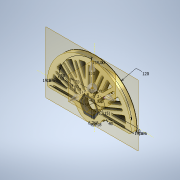
# Autodesk Inventor part: Capstonradialdisc_v2
Saved by Autodesk Inventor 2022 (Build 260153000, 153)
## iProperties
Created: 2022-03-11
Part Number: Capstonradialdisc_v2
Material: Generisch
Document SubType Name: Modeling
Designer: 123St
Density: 1 g/cm^3
Appearance: Gold - Metall
Mass: 270.626 g
Surface Area: 814.649 cm^2
Volume: 270.626 cm^3
CapstonDisc_Thickness: 16,000 mm
CapstonBig_Radius: 120,000 mm
Author: 123St
Autodesk Inventor part; units mm, degrees
ref_plane "YZ Plane" through (0, 0, 0) normal (1, 0, 0) x (0, 1, 0)
ref_plane "XZ Plane" through (0, 0, 0) normal (0, 1, 0) x (-1, 0, 0)
ref_plane "XY Plane" through (0, 0, 0) normal (0, 0, 1) x (1, 0, 0)
sketch "Skizze1" plane through (0, 0, 0) normal (0, 0, 1) x (1, 0, 0)
  line L0 (-4, 29) -> (4, 29)
  line L1 (4, 29) -> (4, 19.5959)
  line L2 (-4, 19.5959) -> (-4, 29)
  line L3 (-4, 29) -> (4, 19.5959) construction
  line L4 (4, 29) -> (-4, 19.5959) construction
  line L5 (0, 152) -> (0, -72) construction
  line L6 (-168, 0) -> (168, 0) construction
  line L7 (-40, 0) -> (-100, 0) construction
  line L8 (-40, -3) -> (-100, -3)
  line L9 (-100, 3) -> (-40, 3)
  arc A0 (-40, -3) -> (-40, 3) centre (-40, 0) ccw
  arc A1 (-100, 3) -> (-100, -3) centre (-100, 0) ccw
  arc A2 (-38.7298, -10) -> (38.7298, -10) centre (0, 0) ccw
  line L10 (-38.7298, -10) -> (-119.5826, -10)
  line L11 (38.7298, -10) -> (119.5826, -10)
  arc A3 (119.5826, -10) -> (-119.5826, -10) centre (0, 0) ccw
  arc A4 (-38.1032, 12.5357) -> (-35.8071, 18.079) centre (-36.9552, 15.3073) ccw
  line L12 (-91.2399, 41.04) -> (-35.8071, 18.079)
  line L13 (-36.9552, 15.3073) -> (-92.388, 38.2683) construction
  arc A5 (-91.2399, 41.04) -> (-93.536, 35.4967) centre (-92.388, 38.2683) ccw
  line L14 (-38.1032, 12.5357) -> (-93.536, 35.4967)
  arc A6 (-30.4056, 26.163) -> (-26.163, 30.4056) centre (-28.2843, 28.2843) ccw
  line L15 (-68.5894, 72.832) -> (-26.163, 30.4056)
  line L16 (-28.2843, 28.2843) -> (-70.7107, 70.7107) construction
  arc A7 (-68.5894, 72.832) -> (-72.832, 68.5894) centre (-70.7107, 70.7107) ccw
  line L17 (-30.4056, 26.163) -> (-72.832, 68.5894)
  arc A8 (-18.079, 35.8071) -> (-12.5357, 38.1032) centre (-15.3073, 36.9552) ccw
  line L18 (-35.4967, 93.536) -> (-12.5357, 38.1032)
  line L19 (-15.3073, 36.9552) -> (-38.2683, 92.388) construction
  arc A9 (-35.4967, 93.536) -> (-41.04, 91.2399) centre (-38.2683, 92.388) ccw
  line L20 (-18.079, 35.8071) -> (-41.04, 91.2399)
  arc A10 (-3, 40) -> (3, 40) centre (0, 40) ccw
  line L21 (3, 100) -> (3, 40)
  line L22 (0, 40) -> (0, 100) construction
  arc A11 (3, 100) -> (-3, 100) centre (0, 100) ccw
  line L23 (-3, 40) -> (-3, 100)
  arc A12 (12.5357, 38.1032) -> (18.079, 35.8071) centre (15.3073, 36.9552) ccw
  line L24 (41.04, 91.2399) -> (18.079, 35.8071)
  line L25 (15.3073, 36.9552) -> (38.2683, 92.388) construction
  arc A13 (41.04, 91.2399) -> (35.4967, 93.536) centre (38.2683, 92.388) ccw
  line L26 (12.5357, 38.1032) -> (35.4967, 93.536)
  arc A14 (26.163, 30.4056) -> (30.4056, 26.163) centre (28.2843, 28.2843) ccw
  line L27 (72.832, 68.5894) -> (30.4056, 26.163)
  line L28 (28.2843, 28.2843) -> (70.7107, 70.7107) construction
  arc A15 (72.832, 68.5894) -> (68.5894, 72.832) centre (70.7107, 70.7107) ccw
  line L29 (26.163, 30.4056) -> (68.5894, 72.832)
  arc A16 (35.8071, 18.079) -> (38.1032, 12.5357) centre (36.9552, 15.3073) ccw
  line L30 (93.536, 35.4967) -> (38.1032, 12.5357)
  line L31 (36.9552, 15.3073) -> (92.388, 38.2683) construction
  arc A17 (93.536, 35.4967) -> (91.2399, 41.04) centre (92.388, 38.2683) ccw
  line L32 (35.8071, 18.079) -> (91.2399, 41.04)
  arc A18 (40, 3) -> (40, -3) centre (40, 0) ccw
  line L33 (100, -3) -> (40, -3)
  line L34 (40, 0) -> (100, 0) construction
  arc A19 (100, -3) -> (100, 3) centre (100, 0) ccw
  line L35 (40, 3) -> (100, 3)
  line L36 (-55.3007, 11) -> (-101.4947, 30.1342)
  line L37 (-101.4947, 30.1342) -> (-105.3007, 11)
  line L38 (-105.3007, 11) -> (-55.3007, 11)
  line L39 (-82.1538, 66.7832) -> (-93.0127, 50.5755)
  line L40 (-46.8426, 31.3838) -> (-82.1538, 66.7832)
  line L41 (-93.0127, 50.5755) -> (-46.8426, 31.3838)
  line L42 (-50.2273, 93.2012) -> (-66.4754, 82.403)
  line L43 (-31.2084, 46.9597) -> (-50.2273, 93.2012)
  line L44 (-66.4754, 82.403) -> (-31.2084, 46.9597)
  line L45 (-10.6061, 105.3411) -> (-29.7544, 101.6067)
  line L46 (-10.7931, 55.3415) -> (-10.6061, 105.3411)
  line L47 (-29.7544, 101.6067) -> (-10.7931, 55.3415)
  line L48 (30.6399, 101.3432) -> (11.525, 105.2446)
  line L49 (11.2756, 55.2452) -> (30.6399, 101.3432)
  line L50 (11.525, 105.2446) -> (11.2756, 55.2452)
  line L51 (67.192, 81.8198) -> (51.0387, 92.7593)
  line L52 (31.617, 46.6855) -> (67.192, 81.8198)
  line L53 (51.0387, 92.7593) -> (31.617, 46.6855)
  line L54 (93.4505, 49.7619) -> (82.7335, 66.0637)
  line L55 (47.1147, 30.9738) -> (93.4505, 49.7619)
  line L56 (82.7335, 66.0637) -> (47.1147, 30.9738)
  line L57 (105.3927, 10.0807) -> (101.7538, 29.2473)
  line L58 (55.3946, 10.517) -> (105.3927, 10.0807)
  line L59 (101.7538, 29.2473) -> (55.3946, 10.517)
  circle A20 centre (0, 0) radius 20
  line L60 (0, 20) -> (4, 20) construction
  line L61 (-4, -29) -> (4, -29)
  line L62 (4, -29) -> (4, -19.5959)
  line L63 (-4, -19.5959) -> (-4, -29)
  line L64 (-4, -29) -> (4, -19.5959) construction
  line L65 (4, -29) -> (-4, -19.5959) construction
  line L66 (0, -20) -> (4, -20) construction
  arc A21 (-4, 19.5959) -> (-4, -19.5959) centre (0, 0) ccw
  arc A22 (4, -19.5959) -> (4, 19.5959) centre (0, 0) ccw
  line L67 (-8.7178, -18) -> (8.7178, -18)
  line L68 (-8.7178, 18) -> (8.7178, 18)
  line L69 (-14.5, -25.1147) -> (-29, 0)
  line L70 (-29, 0) -> (-14.5, 25.1147)
  line L71 (-14.5, 25.1147) -> (14.5, 25.1147)
  line L72 (14.5, 25.1147) -> (29, 0)
  line L73 (29, 0) -> (14.5, -25.1147)
  line L74 (14.5, -25.1147) -> (-14.5, -25.1147)
  line L75 (8.594, -25.1147) -> (26.047, 5.1147) construction
  circle A23 centre (0, 0) radius 29 construction
  point P0 (0, 24.298)
  point P1 (-70, 0)
  point P2 (-64.6716, 26.7878)
  point P3 (-49.4975, 49.4975)
  point P4 (-26.7878, 64.6716)
  point P5 (0, 70)
  point P6 (26.7878, 64.6716)
  point P7 (49.4975, 49.4975)
  point P8 (64.6716, 26.7878)
  point P9 (70, 0)
  point P10 (0, -24.298)
  point P11 (4, -19.5959)
  point P12 (-4, -19.5959)
  point P13 (0, 110)
  point P14 (0, 37)
  point P15 (-8.7178, 18)
  point P16 (8.7178, 18)
  dimension "d67" = 58
  dimension "d2" = 8
  dimension "d7" = 60
  dimension "d8" = 3
  dimension "d9" = 70
  dimension "d12" = 180
  dimension "CapstonBig_Radius" = 120
  dimension "d19" = 40
  dimension "d21" = 8
  dimension "d22" = 8
  dimension "d23" = 50
  dimension "d24" = 50
  dimension "d27" = 158
  dimension "d43" = 20
  dimension "d44" = 10
  dimension "d45" = 110
  dimension "d53" = 2
  dimension "d54" = 8
  dimension "d55" = 18
  dimension "d56" = 8.7178
  dimension "d57" = 19.5959
  dimension "d58" = 4
  dimension "d59" = 19.5959
  dimension "d60" = 4
  dimension "d61" = 18
  dimension "d62" = 8.7178
  dimension "d63" = 2
  dimension "d68" = 5.1147
  constraints: 166 end point, 51 point on circle, 23 centre point, 10 point on line, 8 coincident, 7 parallel, 7 symmetric about line, 7 tangent, 5 midpoint, 4 horizontal, 2 perpendicular, 1 horizontal alignment, 162 other
  measures "d2" distance of L0.start L0.end
  measures "d7" distance of L9.start L9.end
  measures "d8" radius of A0
  measures "d9" distance of point (0, 0) point (-70, 0)
  measures "CapstonBig_Radius" radius of A3
  measures "d19" radius of A2
  measures "d21" distance between parallel lines of L9 L38
  measures "d22" distance between parallel lines of L14 L36
  measures "d23" distance of L37.end L36.start
  measures "d24" distance of L36.start L36.end
  measures "d43" radius of A22
  measures "d44" distance between parallel lines of L11 L6
  measures "d45" distance of point (0, 0) point (0, 110)
  measures "d53" distance from line of L67 L66.start
  measures "d54" distance from line of point (0, 37) L0
  measures "d55" distance from line of point (8.718, -18) L6
  measures "d56" distance from line of point (8.718, -18) L5
  measures "d57" distance from line of point (4, -19.596) L6
  measures "d58" distance from line of point (4, -19.596) L5
  measures "d59" distance from line of point (-4, -19.596) L6
  measures "d60" distance from line of point (-4, -19.596) L5
  measures "d61" distance from line of point (-8.718, -18) L6
  measures "d62" distance from line of point (-8.718, -18) L5
  measures "d63" distance from line of L68 L60.start
  measures "d68" distance between parallel lines of L73 L75
extrude "Extrusion1" add sketch "Skizze1" along normal blind 16 contours L0 L1 L71 L2 | L74 L62 L61 L63 | L10 A3 L11 A2
fillet "Rundung1" radius 15 2 edges at (-38.7298, -10, 8) (38.7298, -10, 8)
fillet "Rundung2" radius 5 2 edges at (119.5826, -10, 8) (-119.5826, -10, 8)
sketch "Skizze2" plane through (48.9898, -10, 0) normal (0, -1, 0) x (1, 0, 0)
  circle A0 centre (62.8967, 4) radius 1
  line L0 (0, 0) -> (65.9015, 0) projected
  circle A1 centre (-160.8763, 12) radius 1
  line L1 (-163.881, 16) -> (-97.9796, 16) projected
  line L2 (-168.8763, 16) -> (-168.8763, 0) projected
  line L3 (70.8967, 0) -> (70.8967, 16) projected
  point P0 (-48.9898, 0)
  dimension "d29" = 4
  dimension "d30" = 2
  dimension "d31" = 4
  dimension "d32" = 2
  dimension "d33" = 8
  dimension "d34" = 8
  constraints: 2 centre point
  measures "d29" distance from line of L0 A0.centre
  measures "d30" diameter of A0
  measures "d31" distance from line of L1 A1.centre
  measures "d32" diameter of A1
  measures "d33" distance from line of L2 A1.centre
  measures "d34" distance from line of L3 A0.centre
extrude "Extrusion2" cut sketch "Skizze2" against normal blind 15
fillet "Rundung3" radius 2 24 edges at (-101.4947, 30.1342, 8) (-105.3007, 11, 8) (-93.0127, 50.5755, 8) (-66.4754, 82.403, 8) (-10.6061, 105.3411, 8) (-50.2273, 93.2012, 8) (-82.1538, 66.7832, 8) (-29.7544, 101.6067, 8) (30.6399, 101.3432, 8) (11.525, 105.2446, 8) (67.192, 81.8198, 8) (51.0387, 92.7593, 8) (93.4505, 49.7619, 8) (82.7335, 66.0637, 8) (101.7538, 29.2473, 8) (105.3927, 10.0807, 8) (-55.3007, 11, 8) (-46.8426, 31.3838, 8) (-31.2084, 46.9597, 8) (-10.7931, 55.3415, 8) (11.2756, 55.2452, 8) (31.617, 46.6855, 8) (47.1147, 30.9738, 8) (55.3946, 10.517, 8)
ref_plane "Arbeitsebene1" through (0, 0, 8) normal (0, 0, 1) x (1, 0, 0)
extrude "Extrusion4" add sketch "Skizze1" along normal up to surface (16 mm away) separate body contours L71 L1 A20 L2 | L2 A20 L63 L74 L69 L70 L71 | L71 L72 L73 L74 L62 A20 L1 | L67 A20 | A20 L62 L74 L63
sketch "Sketch3" plane through (-14.5, -25.1147, 16) normal (0, 0, 1) x (1, 0, 0)
  circle A0 centre (5.7822, 7.1147) radius 0.75
  circle A1 centre (23.2178, 7.1147) radius 0.75
  point P0 (14.5, 25.1147)
  dimension "d75" = 1.5
  constraints: 2 centre point, 2 coincident, 1 equal radius
  measures "d75" diameter of A0
extrude "Extrusion5" cut sketch "Sketch3" against normal through all bodies 2
equation "\"d43\" = Shaft_CapstonPart_Dia"
equation "\"Shaft_CapstonPart_Dia\" = 20"
